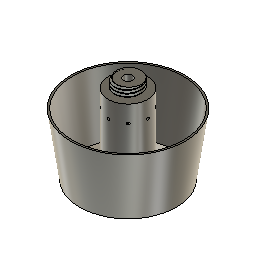
plant (Autodesk Fusion 360 design; units mm, degrees)
Autodesk Fusion 360 part; units mm, degrees
note: some values were not read from the file. Set by a fixed rule: which face or edge a step refers to.
sketch "スケッチ1" plane through (0, 0, 0) normal (0, 0, 1) x (1, 0, 0)
  circle A0 centre (0, 0) radius 55
  dimension "d1" = 110
  constraint coincident A0.centre origin
  measures "d1" diameter of A0
ref_plane "作業平面2" through (0, 0, 70) normal (0, 0, 1) x (1, 0, 0)
sketch "スケッチ2" plane through (0, 0, 70) normal (0, 0, 1) x (1, 0, 0)
  circle A0 centre (0, 0) radius 65
  dimension "d4" = 130
  constraint coincident A0.centre origin
  measures "d4" diameter of A0
loft "ロフト1" add profiles "スケッチ2", "スケッチ1" section 1 section 2
shell "シェル1" thickness 2 removed faces 1 at (-2.3225, 16.9397, 70)
ref_plane "作業平面3" through (0, 0, 20) normal (0, 0, 1) x (1, 0, 0)
sketch "スケッチ3" plane through (0, 0, 20) normal (0, 0, 1) x (1, 0, 0)
  circle A0 centre (0, 0) radius 22.5
  dimension "d7" = 45
  constraint coincident A0.centre origin
  measures "d7" diameter of A0
loft "ロフト2" add profiles "スケッチ3" section 1 section 2 face at (9.655, 2.6463, 2)
extrude "押し出し1" add 1 faces at (2.0784, -12.7768, 20) along direction (0, 0, 1) blind 80
sketch "スケッチ4" plane through (0, 0, 100) normal (0, 0, 1) x (-1, 0, 0)
  circle A0 centre (0, 0) radius 22.5
  circle A1 centre (0, 0) radius 5
  dimension "d10" = 10
  constraint coincident A0.centre A1.centre
  measures "d10" diameter of A1
extrude "押し出し2" cut sketch "スケッチ4" against normal blind 80 contours A1
sketch "スケッチ5" plane through (0, 0, 0) normal (0, 0, -1) x (1, 0, 0)
  circle A0 centre (0, 0) radius 55
  circle A1 centre (0, 0) radius 5
  circle A2 centre (0, 0) radius 7
  circle A3 centre (0, 0) radius 20
  dimension "d13" = 10
  dimension "d14" = 14
  dimension "d15" = 40
  constraint coincident A0.centre A1.centre
  constraint concentric A1 A2
  constraint concentric A1 A3
  measures "d13" diameter of A1
  measures "d14" diameter of A2
  measures "d15" diameter of A3
extrude "押し出し6" cut sketch "スケッチ5" against normal blind 75 contours A3
extrude "押し出し7" add sketch "スケッチ5" against normal blind 60 contours A3
extrude "押し出し8" cut sketch "スケッチ5" against normal blind 100 contours A1
sketch "スケッチ7" plane through (0, 0, 0) normal (0, 0, -1) x (1, 0, 0)
  circle A0 centre (13.32, 0.0717) radius 5.5
  dimension "d29" = 11
  measures "d29" diameter of A0
extrude "押し出し9" cut sketch "スケッチ7" against normal blind 70
ref_plane "作業平面4" through (0, -22.5, 74.8261) normal (0, -1, 0) x (-1, 0, 0)
sketch "スケッチ8" plane through (0, -22.5, 74.8261) normal (0, -1, 0) x (1, 0, 0)
  circle A0 centre (0.1394, -3.9134) radius 1.5
  dimension "d33" = 3
  measures "d33" diameter of A0
extrude "押し出し10" cut sketch "スケッチ8" against normal blind 13
pattern_circular "C パターン1" count 8 over 360 about axis through (0, 0, 1.75) along (0, 0, 1) of 1 faces at (1.0935, -20.8045, 72.0702)
sketch "スケッチ9" plane through (0, 0, 100) normal (0, 0, 1) x (-1, 0, 0)
  circle A0 centre (0, 0) radius 15
  circle A1 centre (0, 0) radius 22.5
  dimension "d38" = 30
  dimension "d39" = 45
  constraint coincident A0.centre A1.centre
  measures "d38" diameter of A0
  measures "d39" diameter of A1
extrude "押し出し11" cut sketch "スケッチ9" against normal blind 10
thread "ねじ1" "ISO Metric profile 30.0 M30x3.5 6g" major diameter 29.7345 minor diameter 25.732 pitch 3.5 angle 60 modelled right hand crest width 0.4992 on face at (-14.9814, 0.7477, 93.3333) crest through (-14.8673, 0, 100.875)
